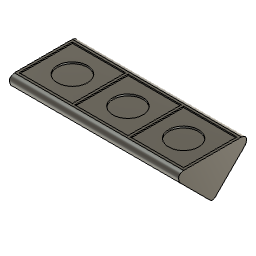
nfc frame (Autodesk Fusion 360 design; units mm, degrees)
Autodesk Fusion 360 part; units mm, degrees
sketch "Sketch1" plane through (0, 0, 0) normal (0, 0, 1) x (1, 0, 0)
  line L0 (0, 0) -> (45, 0)
  line L1 (45, 0) -> (45, 45)
  line L2 (45, 45) -> (0, 45)
  line L3 (0, 45) -> (0, 0)
  line L4 (0, 22.5) -> (0, 0)
  line L5 (0, 0) -> (22.5, 0)
  line L6 (22.5, 0) -> (22.5, 22.5)
  line L7 (22.5, 22.5) -> (0, 22.5)
  line L8 (0, 22.5) -> (0, 0)
  circle A0 centre (22.5, 22.5) radius 12.7
  line L9 (0, 22.5) -> (0, 0)
  line L10 (22.5, 0) -> (22.5, 22.5)
  line L11 (45, 45) -> (0, 45)
  line L12 (45, 0) -> (45, 45)
  line L13 (0, 45) -> (0, 0)
  circle A1 centre (22.5, 22.5) radius 12.7
  line L14 (22.5, 22.5) -> (0, 22.5)
  line L15 (0, 0) -> (45, 0)
  line L16 (0, 22.5) -> (0, 0)
  line L17 (0, 0) -> (22.5, 0)
  line L18 (-2, -2) -> (47, -2)
  line L19 (47, -2) -> (47, 47)
  line L20 (47, 47) -> (-2, 47)
  line L21 (-2, 47) -> (-2, -2)
  line L22 (0, 0) -> (22.5, 0)
  line L23 (47, 47) -> (-2, 47)
  line L24 (-2, 47) -> (-2, -2)
  line L25 (0, 45) -> (0, 0)
  line L26 (22.5, 22.5) -> (0, 22.5)
  line L27 (45, 45) -> (0, 45)
  line L28 (47, -2) -> (47, 47)
  line L29 (0, 0) -> (45, 0)
  line L30 (0, 0) -> (22.5, 0)
  line L31 (22.5, 0) -> (22.5, 22.5)
  line L32 (0, 22.5) -> (0, 0)
  line L33 (45, 0) -> (45, 45)
  line L34 (45, 45) -> (0, 45)
  line L35 (22.5, 22.5) -> (0, 22.5)
  circle A2 centre (22.5, 22.5) radius 12.7
  circle A3 centre (22.5, 22.5) radius 12.7
  line L36 (22.5, 0) -> (22.5, 22.5)
  line L37 (0, 22.5) -> (0, 0)
  line L38 (0, 22.5) -> (0, 0)
  line L39 (0, 0) -> (45, 0)
  line L40 (0, 22.5) -> (0, 0)
  line L41 (0, 45) -> (0, 0)
  line L42 (-2, -2) -> (47, -2)
  line L43 (45, 0) -> (45, 45)
  line L44 (47, 0) -> (69.5, 0)
  line L45 (94, 47) -> (45, 47)
  line L46 (45, 47) -> (45, -2)
  line L47 (47, 45) -> (47, 0)
  line L48 (69.5, 22.5) -> (47, 22.5)
  line L49 (92, 45) -> (47, 45)
  line L50 (94, -2) -> (94, 47)
  line L51 (47, 0) -> (92, 0)
  line L52 (47, 0) -> (69.5, 0)
  line L53 (69.5, 0) -> (69.5, 22.5)
  line L54 (47, 22.5) -> (47, 0)
  line L55 (92, 0) -> (92, 45)
  line L56 (92, 45) -> (47, 45)
  line L57 (69.5, 22.5) -> (47, 22.5)
  circle A4 centre (69.5, 22.5) radius 12.7
  circle A5 centre (69.5, 22.5) radius 12.7
  line L58 (69.5, 0) -> (69.5, 22.5)
  line L59 (47, 22.5) -> (47, 0)
  line L60 (47, 22.5) -> (47, 0)
  line L61 (47, 0) -> (92, 0)
  line L62 (47, 22.5) -> (47, 0)
  line L63 (47, 45) -> (47, 0)
  line L64 (45, -2) -> (94, -2)
  line L65 (92, 0) -> (92, 45)
  line L66 (94, 0) -> (116.5, 0)
  line L67 (141, 47) -> (92, 47)
  line L68 (92, 47) -> (92, -2)
  line L69 (94, 45) -> (94, 0)
  line L70 (116.5, 22.5) -> (94, 22.5)
  line L71 (139, 45) -> (94, 45)
  line L72 (141, -2) -> (141, 47)
  line L73 (94, 0) -> (139, 0)
  line L74 (94, 0) -> (116.5, 0)
  line L75 (116.5, 0) -> (116.5, 22.5)
  line L76 (94, 22.5) -> (94, 0)
  line L77 (139, 0) -> (139, 45)
  line L78 (139, 45) -> (94, 45)
  line L79 (116.5, 22.5) -> (94, 22.5)
  circle A6 centre (116.5, 22.5) radius 12.7
  circle A7 centre (116.5, 22.5) radius 12.7
  line L80 (116.5, 0) -> (116.5, 22.5)
  line L81 (94, 22.5) -> (94, 0)
  line L82 (94, 22.5) -> (94, 0)
  line L83 (94, 0) -> (139, 0)
  line L84 (94, 22.5) -> (94, 0)
  line L85 (94, 45) -> (94, 0)
  line L86 (92, -2) -> (141, -2)
  line L87 (139, 0) -> (139, 45)
  point P0 (47, 0)
  point P1 (47, 0)
  point P2 (94, 0)
  point P3 (94, 0)
  dimension "d1" = 45
  dimension "d2" = 45
  dimension "d14" = 22.5
  dimension "d15" = 25.4
  dimension "d16" = 45
  dimension "d17" = 45
  dimension "d18" = 22.5
  dimension "d19" = 25.4
  dimension "d20" = 45
  dimension "d21" = 45
  dimension "d22" = 22.5
  dimension "d23" = 25.4
  dimension "d24" = 45
  dimension "d25" = 45
  dimension "d26" = 22.5
  dimension "d27" = 25.4
  dimension "d28" = 45
  dimension "d29" = 45
  dimension "d30" = 22.5
  dimension "d31" = 25.4
  dimension "d32" = 45
  dimension "d33" = 45
  dimension "d34" = 22.5
  dimension "d35" = 25.4
  dimension "d36" = 45
  dimension "d37" = 45
  dimension "d38" = 22.5
  dimension "d39" = 25.4
  dimension "d40" = 45
  dimension "d41" = 45
  dimension "d42" = 22.5
  dimension "d43" = 25.4
  constraint horizontal L0
  constraint vertical L1
  constraint horizontal L2
  constraint vertical L3
  constraint coincident L0.start L3.end
  constraint vertical L4
  constraint horizontal L5
  constraint vertical L6
  constraint horizontal L7
  constraint vertical L8
  constraint coincident L6.end L7.start
  constraint horizontal L15
  constraint vertical L12
  constraint horizontal L11
  constraint vertical L13
  constraint vertical L16
  constraint horizontal L17
  constraint vertical L10
  constraint horizontal L14
  constraint vertical L9
  constraint horizontal L18
  constraint vertical L19
  constraint horizontal L20
  constraint vertical L21
  constraint horizontal L29
  constraint vertical L33
  constraint horizontal L27
  constraint vertical L25
  constraint vertical L37
  constraint horizontal L30
  constraint vertical L31
  constraint horizontal L26
  constraint vertical L38
  constraint horizontal L39
  constraint vertical L43
  constraint horizontal L34
  constraint vertical L41
  constraint vertical L32
  constraint horizontal L22
  constraint vertical L36
  constraint horizontal L35
  constraint vertical L40
  constraint horizontal L42
  constraint vertical L28
  constraint horizontal L23
  constraint vertical L24
  constraint horizontal L51
  constraint vertical L55
  constraint horizontal L49
  constraint vertical L47
  constraint coincident P1 P0
  constraint vertical L59
  constraint horizontal L52
  constraint vertical L53
  constraint horizontal L48
  constraint vertical L60
  constraint coincident L48.start L53.end
  constraint horizontal L61
  constraint vertical L65
  constraint horizontal L56
  constraint vertical L63
  constraint vertical L54
  constraint horizontal L44
  constraint vertical L58
  constraint horizontal L57
  constraint vertical L62
  constraint horizontal L64
  constraint vertical L50
  constraint horizontal L45
  constraint vertical L46
  constraint horizontal L73
  constraint vertical L77
  constraint horizontal L71
  constraint vertical L69
  constraint coincident P3 P2
  constraint vertical L81
  constraint horizontal L74
  constraint vertical L75
  constraint horizontal L70
  constraint vertical L82
  constraint coincident L70.start L75.end
  constraint horizontal L83
  constraint vertical L87
  constraint horizontal L78
  constraint vertical L85
  constraint vertical L76
  constraint horizontal L66
  constraint vertical L80
  constraint horizontal L79
  constraint vertical L84
  constraint horizontal L86
  constraint vertical L72
  constraint horizontal L67
  constraint vertical L68
  measures "d1" distance of L0.start L0.end
  measures "d2" distance of L0.start L2.end
  measures "d14" distance of L0.start L5.end
  measures "d15" diameter of A0
  measures "d16" distance of L0.start L0.end
  measures "d17" distance of L0.start L2.end
  measures "d18" distance of L0.start L5.end
  measures "d19" diameter of A1
  measures "d20" distance of L0.start L0.end
  measures "d21" distance of L0.start L2.end
  measures "d22" distance of L5.end L0.start
  measures "d23" diameter of A3
  measures "d24" distance of L0.start L0.end
  measures "d25" distance of L0.start L2.end
  measures "d26" distance of L0.start L5.end
  measures "d27" diameter of A2
  measures "d28" distance of P1 L51.end
  measures "d29" distance of P1 L47.start
  measures "d30" distance of L44.end P1
  measures "d31" diameter of A5
  measures "d32" distance of P1 L51.end
  measures "d33" distance of P1 L47.start
  measures "d34" distance of P1 L44.end
  measures "d35" diameter of A4
  measures "d36" distance of P3 L73.end
  measures "d37" distance of P3 L69.start
  measures "d38" distance of L66.end P3
  measures "d39" diameter of A7
  measures "d40" distance of P3 L73.end
  measures "d41" distance of P3 L69.start
  measures "d42" distance of P3 L66.end
  measures "d43" diameter of A6
extrude "Extrude5" add sketch "Sketch1" along normal blind 2 contours L6 L7 A0 L10 A1 L14 L26 L31 L35 A2 A3 L36 | L6 L7 A0 L10 A1 L14 L26 L31 L35 A2 A3 L36 | L48 L53 L57 A4 A5 L58 | L48 L53 L57 A4 A5 L58 | L70 L75 L79 A6 A7 L80 | L70 L75 L79 A6 A7 L80 makes body 1 at (24.1974, 23.3174, 2) makes body 2 at (65.7084, 17.8668, 0) makes body 3 at (114.0114, 16.3661, 0)
extrude "Extrude6" add sketch "Sketch1" along normal blind 3.4 contours L0 L3 L4 L5 L6 L7 L8 A0 L9 L10 L13 A1 L14 L15 L16 L17 L22 L25 L26 L29 L30 L31 L32 L35 A2 A3 L36 L37 L38 L39 L40 L41 | L0 L1 L2 L3 L6 L7 A0 L10 L11 L12 L13 A1 L14 L15 L25 L26 L27 L29 L31 L33 L34 L35 A2 A3 L36 L39 L41 L43 L46 | L19 L28 L44 L47 L48 L51 L52 L53 L54 L57 A4 A5 L58 L59 L60 L61 L62 L63 | L19 L28 L47 L48 L49 L51 L53 L55 L56 L57 A4 A5 L58 L61 L63 L65 L68 | L50 L66 L69 L70 L73 L74 L75 L76 L79 A6 A7 L80 L81 L82 L83 L84 L85 | L50 L69 L70 L71 L73 L75 L77 L78 L79 A6 A7 L80 L83 L85 L87 bodies 1 2 3
extrude "Extrude7" add sketch "Sketch1" along normal blind 4.4 contours L0 L2 L3 L4 L5 L8 L9 L11 L13 L15 L16 L17 L18 L20 L21 L22 L23 L24 L25 L27 L29 L30 L32 L34 L37 L38 L39 L40 L41 L42 L46 | L1 L12 L18 L19 L20 L23 L28 L33 L42 L43 L45 L46 L47 L54 L59 L60 L62 L63 L64 | L19 L28 L44 L51 L52 L61 L64 L68 | L19 L28 L45 L49 L56 L68 | L45 L50 L55 L64 L65 L67 L68 L69 L76 L81 L82 L84 L85 L86 | L50 L66 L67 L71 L72 L73 L74 L77 L78 L83 L86 L87 bodies 1 2 3
sketch "Sketch2" plane through (-2, 0, 0) normal (-1, 0, 0) x (0, -1, 0)
  line L0 (-47, 0) -> (2, 0)
  line L1 (2, 0) -> (2, 4.4)
  line L2 (2, 4.4) -> (-47, 4.4)
  line L3 (-47, 4.4) -> (-47, 0)
  line L4 (-47, 0) -> (-18.7157, -28.2843)
  line L5 (-47, 0) -> (-7, 0) construction
  line L6 (2, 0) -> (-26.2843, -28.2843)
  line L7 (2, 0) -> (42, 0) construction
  line L8 (2, 0) -> (5.1113, -3.1113)
  line L9 (2, 0) -> (6.4, 0) construction
  line L10 (5.1113, -3.1113) -> (-27.2069, -35.4294)
  line L11 (-47, 0) -> (-50.1113, -3.1113)
  line L12 (-50.1113, -3.1113) -> (-19.4672, -33.7553)
  spline S0 degree 5 poles (-50.1113, -3.1113) (-50.2357, -2.8651) (-50.4685, -2.381) (-50.7692, -1.6797) (-51.0717, -0.7953) (-51.2745, 0.2201) (-51.2858, 1.1369) (-51.089, 1.9469) (-50.6737, 2.6444) (-50.0463, 3.2329) (-49.2221, 3.7203) (-48.4178, 4.0356) (-47.7381, 4.2328) (-47.2516, 4.3471) (-47, 4.4) knots 0 0 0 0 0 0 0.1 0.2 0.3 0.4 0.5 0.6 0.7 0.8 0.9 1 1 1 1 1 1
  spline S1 degree 5 poles (5.1113, -3.1113) (5.2357, -2.8651) (5.4685, -2.381) (5.7692, -1.6797) (6.0717, -0.7953) (6.2745, 0.2201) (6.2858, 1.1369) (6.089, 1.9469) (5.6737, 2.6444) (5.0463, 3.2329) (4.2221, 3.7203) (3.4178, 4.0356) (2.7381, 4.2328) (2.2516, 4.3471) (2, 4.4) knots 0 0 0 0 0 0 0.1 0.2 0.3 0.4 0.5 0.6 0.7 0.8 0.9 1 1 1 1 1 1
  point P0 (-51, 2)
  point P1 (6, 2)
  dimension "d50" = 40
  dimension "d51" = 45
  dimension "d52" = 135
  dimension "d53" = 40
  dimension "d54" = 4.4
  dimension "d55" = 45
  dimension "d56" = 4.4
  constraint horizontal L5
  constraint coincident L0.start L3.end
  constraint horizontal L7
  constraint coincident L0.end L1.start
  constraint horizontal L9
  constraint perpendicular L4 L10
  constraint perpendicular L4 L11
  constraint perpendicular L10 L12
  constraint coincident L2.end L3.start
  constraint coincident L1.end L2.start
  measures "d50" distance of L0.start L4.end
  measures "d51" angle of L4 L5
  measures "d52" angle of L6 L7
  measures "d53" distance of L0.end L6.end
  measures "d54" distance of L0.end L8.end
  measures "d55" angle of L8 L9
  measures "d56" distance of L0.start L11.end
extrude "Extrude8" add sketch "Sketch2" against normal blind 143 contours L3 L11 S0 | L0 L4 L6 | L4 L6 L11 L12 | L4 L6 L8 L10 | L1 L8 S1 | L4 L6 L10 L12 bodies 1
fillet "Fillet1" radius 3 1 edges at (69.5, 22.5, -30.7225) on bodies 1
